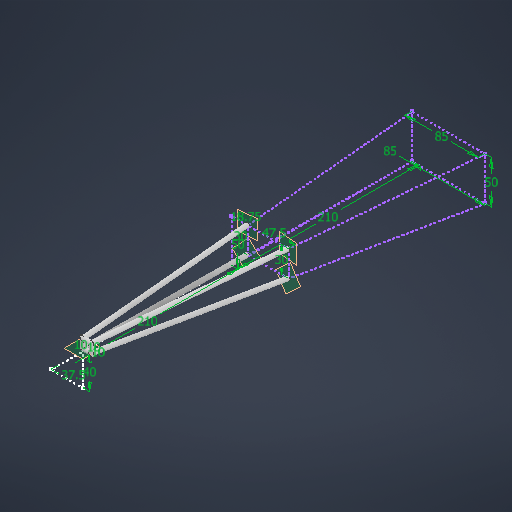
# Autodesk Inventor part: RCPlaneTailRear2
Saved by Autodesk Inventor 2026.1 (Build 301233000, 233)
## iProperties
Created: 2026-03-16
Part Number: RCPlaneTailRear2
Material: Generic
Document SubType Name: Modeling
Designer: morri
Density: 1 g/cm^3
Appearance: Default
Mass: 17.3815 g
Surface Area: 140.623 cm^2
Volume: 17.3815 cm^3
Author: morri
Autodesk Inventor part; units mm, degrees
ref_plane "YZ Plane" through (0, 0, 0) normal (1, 0, 0) x (0, 1, 0)
ref_plane "XZ Plane" through (0, 0, 0) normal (0, 1, 0) x (-1, 0, 0)
ref_plane "XY Plane" through (0, 0, 0) normal (0, 0, 1) x (1, 0, 0)
sketch3d "3D Sketch1"
ref_plane "Work Plane1" through (18.75, 50, 210) normal (-0.0889, 0, -0.996) x (0, -1, 0)
ref_plane "Work Plane2" through (66.25, 20, 210) normal (0.0885, -0.0944, -0.9916) x (0.7295, 0.6839, 0)
ref_plane "Work Plane3" through (66.25, 50, 210) normal (0.0889, 0, -0.996) x (0, 1, 0)
ref_plane "Work Plane4" through (18.75, 20, 210) normal (-0.0885, -0.0944, -0.9916) x (0.7295, -0.6839, 0)
ref_plane "Work Plane5" through (37.5, 40, 420) normal (0, -1, 0) x (1, 0, 0)
sketch "Sketch1" plane through (18.75, 20, 210) normal (-0.0885, -0.0944, -0.9916) x (0.7295, -0.6839, 0)
  circle A0 centre (0, 0) radius 2.5
  point P0 (0, 0)
  dimension "d15" = 5
  constraints: 1 centre point, 1 coincident
  measures "d15" diameter of A0
sketch "Sketch2" plane through (18.75, 50, 210) normal (-0.0889, 0, -0.996) x (0, -1, 0)
  circle A0 centre (0, 0) radius 2.5
  point P0 (50, 0)
  dimension "d16" = 5
  constraints: 1 centre point
  measures "d16" diameter of A0
sketch "Sketch3" plane through (66.25, 50, 210) normal (0.0889, 0, -0.996) x (0, 1, 0)
  circle A0 centre (0, 0) radius 2.5
  point P0 (-50, -84.6632)
  dimension "d17" = 5
  constraints: 1 centre point
  measures "d17" diameter of A0
sketch "Sketch4" plane through (66.25, 20, 210) normal (0.0885, -0.0944, -0.9916) x (0.7295, 0.6839, 0)
  circle A0 centre (0, 0) radius 2.5
  point P0 (-62.0107, -57.6459)
  dimension "d18" = 5
  constraints: 1 centre point
  measures "d18" diameter of A0
sketch "Sketch5" plane through (37.5, 40, 420) normal (0, -1, 0) x (1, 0, 0)
  circle A0 centre (0, 0) radius 2.5
  point P0 (-37.5, -420)
  dimension "d19" = 5
  constraints: 1 centre point
  measures "d19" diameter of A0
sketch3d "3D Sketch2"
  line L0 (18.75, 20, 210) -> (37.5, 40, 420)
  dimension "d9" = 210
  dimension "d10" = 37.5
  dimension "d11" = 40
  dimension "d12" = 10
  dimension "d13" = 10
  dimension "d14" = 10
sweep "Sweep1" add profiles "Sketch1" path "3D Sketch2"
sketch3d "3D Sketch2 for Sweep2"
  line L0 (18.75, 50, 210) -> (37.5, 50, 420)
  dimension "d9" = 210
  dimension "d10" = 37.5
  dimension "d11" = 40
  dimension "d12" = 10
  dimension "d13" = 10
  dimension "d14" = 10
sweep "Sweep2" add profiles "Sketch2" path "3D Sketch2 for Sweep2" separate body
sketch3d "3D Sketch2 for Sweep3"
  line L0 (66.25, 50, 210) -> (47.5, 50, 420)
  dimension "d9" = 210
  dimension "d10" = 37.5
  dimension "d11" = 40
  dimension "d12" = 10
  dimension "d13" = 10
  dimension "d14" = 10
sweep "Sweep3" add profiles "Sketch3" path "3D Sketch2 for Sweep3" separate body
sketch3d "3D Sketch2 for Sweep4"
  line L0 (66.25, 20, 210) -> (47.5, 40, 420)
  dimension "d9" = 210
  dimension "d10" = 37.5
  dimension "d11" = 40
  dimension "d12" = 10
  dimension "d13" = 10
  dimension "d14" = 10
sweep "Sweep4" add profiles "Sketch4" path "3D Sketch2 for Sweep4" separate body
sketch3d "3D Sketch2 for Sweep5"
  line L0 (37.5, 40, 420) -> (37.5, 50, 420)
  line L1 (37.5, 50, 420) -> (47.5, 50, 420)
  line L2 (47.5, 50, 420) -> (47.5, 40, 420)
  line L3 (47.5, 40, 420) -> (37.5, 40, 420)
  dimension "d9" = 210
  dimension "d10" = 37.5
  dimension "d11" = 40
  dimension "d12" = 10
  dimension "d13" = 10
  dimension "d14" = 10
sweep "Sweep5" add profiles "Sketch5" path "3D Sketch2 for Sweep5" separate body
body "Solid1"
body "Solid2"
body "Solid3"
body "Solid4"
body "Solid5"
